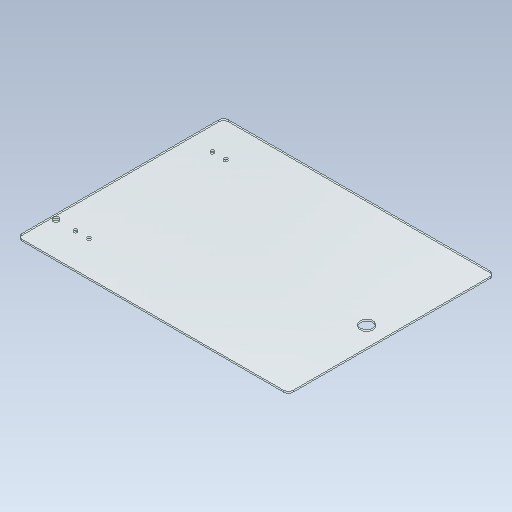
# Autodesk Inventor part: Puerta Frontal
Saved by Autodesk Inventor 2020 (Build 240168000, 168)
## iProperties
Created: 2020-06-12
Part Number: Puerta Frontal
Material: Genérico
Document SubType Name: Modeling
Designer: Pipi
Density: 1 g/cm^3
Appearance: Claro
Author: Pipi
Autodesk Inventor part; units mm, degrees
ref_plane "YZ Plane" through (0, 0, 0) normal (1, 0, 0) x (0, 1, 0)
ref_plane "XZ Plane" through (0, 0, 0) normal (0, 1, 0) x (-1, 0, 0)
ref_plane "XY Plane" through (0, 0, 0) normal (0, 0, 1) x (1, 0, 0)
sketch "Boceto1" plane through (0, 0, 0) normal (0, 1, 0) x (-1, 0, 0)
  line L0 (458.528, 57.3975) -> (70.528, 57.3975)
  line L1 (63.528, 64.3975) -> (63.528, 356.3975)
  line L2 (70.528, 363.3975) -> (458.528, 363.3975)
  line L3 (465.528, 356.3975) -> (465.528, 64.3975)
  circle A0 centre (410.528, 311.6475) radius 2.5
  circle A1 centre (410.528, 109.1475) radius 2.5
  circle A2 centre (430.528, 109.1475) radius 2.5
  circle A3 centre (430.528, 311.6475) radius 2.5
  circle A4 centre (459.528, 311.6475) radius 4
  circle A5 centre (93.528, 217.3975) radius 9.5
  line L4 (69.9652, 363.3975) -> (70.528, 363.3975)
  line L5 (63.528, 355.5516) -> (63.528, 356.3975)
  line L6 (63.528, 65.3975) -> (63.528, 64.3975)
  line L7 (71.528, 57.3975) -> (70.528, 57.3975)
  line L8 (465.528, 65.3975) -> (465.528, 64.3975)
  arc A6 (458.528, 57.3975) -> (465.528, 64.3975) centre (458.528, 64.3975) ccw
  arc A7 (63.528, 64.3975) -> (70.528, 57.3975) centre (70.528, 64.3975) ccw
  arc A8 (70.528, 363.3975) -> (63.528, 356.3975) centre (70.528, 356.3975) ccw
  arc A9 (465.528, 356.3975) -> (458.528, 363.3975) centre (458.528, 356.3975) ccw
  point P0 (0, 0)
  point P1 (457.528, 57.3975)
  point P2 (465.528, 363.3975)
  point P3 (465.528, 57.3975)
  point P4 (63.528, 57.3975)
  point P5 (63.528, 363.3975)
  dimension "d11" = 306
  dimension "d14" = 402
  dimension "d15" = 5
  dimension "d16" = 55
  dimension "d17" = 51.75
  dimension "d18" = 5
  dimension "d19" = 55
  dimension "d20" = 202.5
  dimension "d21" = 5
  dimension "d22" = 20
  dimension "d23" = 5
  dimension "d24" = 20
  dimension "d25" = 8
  dimension "d26" = 6
  dimension "d28" = 19
  dimension "d29" = 30
  dimension "d30" = 51.75
  dimension "d33" = 7
  dimension "d34" = 7
  dimension "d35" = 146
  constraints: 18 end point, 18 point on line, 10 centre point, 8 point on circle, 8 tangent, 5 vertical, 2 equal radius, 2 horizontal
  measures "d11" distance between parallel lines of L2 L0
  measures "d14" distance between parallel lines of L1 L3
  measures "d15" diameter of A0
  measures "d16" distance from line of L3 A0.centre
  measures "d17" distance from line of L2 A0.centre
  measures "d18" diameter of A1
  measures "d19" distance from line of L3 A1.centre
  measures "d20" distance of A0.centre A1.centre
  measures "d21" diameter of A2
  measures "d22" distance of A1.centre A2.centre
  measures "d23" diameter of A3
  measures "d24" distance of A0.centre A3.centre
  measures "d25" diameter of A4
  measures "d26" distance from line of L3 A4.centre
  measures "d28" diameter of A5
  measures "d29" distance from line of A5.centre L1
  measures "d30" distance from line of A4.centre L2
  measures "d33" radius of A6
  measures "d34" radius of A7
  measures "d35" distance from line of L2 A5.centre
extrude "Extrusión1" add sketch "Boceto1" along normal blind 2.4
